Autodesk Fusion 360 part; units mm, degrees
(part 4 of 5)
sketch "Sketch2" plane through (0, 0, 0) normal (0, 0, 1) x (1, 0, 0)
  arc A0 (28.2898, -146.7842) -> (30.0064, -147.0869) centre (30.8779, -137.1249) ccw construction
  arc A1 (9.3424, -112.1265) -> (12.7274, -116.0513) centre (22.2229, -104.4394) ccw construction
  line L0 (9.8518, -167.6702) -> (17.4021, -163.8233) construction
  circle A2 centre (2.1789, -108.5649) radius 3.375 construction
  line L1 (100.4519, -39.9064) -> (12.7274, -116.0513) construction
  line L2 (28.2898, -146.7842) -> (23.615, -145.5316) construction
  arc A3 (30.9564, -136.2283) -> (29.2133, -136.2283) centre (30.0848, -146.1903) ccw construction
  arc A4 (2.3786, -152.7505) -> (5.279, -154.7068) centre (4.371, -152.9248) ccw construction
  arc A5 (100.4519, -39.9064) -> (105.7604, -37.9868) centre (99.4908, -28.9484) ccw construction
  line L3 (18.4399, -134.3914) -> (17.361, -146.7224) construction
  line L4 (22.8776, -144.4785) -> (23.4829, -137.5592) construction
  arc A6 (-11.1082, -168.6356) -> (3.7484, -173.4033) centre (-3.1387, -169.3329) ccw construction
  arc A7 (23.3547, -162.6662) -> (17.4021, -163.8233) centre (22.396, -173.6243) ccw construction
  line L5 (-5.7907, -107.8678) -> (-7.6374, -128.9799)
  arc A8 (-9.2616, -147.5287) -> (-11.8245, -142.975) centre (-13.8718, -147.1253) ccw construction
  line L6 (4.7746, -145.5276) -> (6.1209, -144.398) construction
  line L7 (24.392, -136.6501) -> (29.2133, -136.2283) construction
  arc A9 (-10.9528, -133.0126) -> (-7.6374, -128.9799) centre (-12.2491, -128.5675) ccw
  circle A10 centre (27.1493, -126.0578) radius 1.5 construction
  line L8 (6.9668, -134.7286) -> (5.8373, -133.3824) construction
  line L9 (-9.2616, -147.5287) -> (-11.1082, -168.6356) construction
  arc A11 (22.8776, -144.4785) -> (23.615, -145.5316) centre (23.8738, -144.5656) ccw construction
  circle A12 centre (24.4911, -156.4418) radius 1.5 construction
  arc A13 (7.9279, -124.4303) -> (4.7319, -125.8533) centre (6.7243, -126.0276) ccw construction
  arc A14 (9.8518, -167.6702) -> (3.7484, -173.4033) centre (16.6616, -181.0354) ccw construction
  circle A15 centre (-3.7013, -153.9753) radius 1.5 construction
  arc A16 (9.3424, -112.1265) -> (-5.7907, -107.8678) centre (2.1789, -108.5649) ccw construction
  arc A17 (24.392, -136.6501) -> (23.4829, -137.5592) centre (24.4791, -137.6463) ccw construction
  line L10 (15.7692, -149.4168) -> (5.279, -154.7068) construction
  line L11 (2.3786, -152.7505) -> (2.6542, -149.601) construction
  circle A18 centre (31.9218, -131.7454) radius 1.5 construction
  line L12 (7.9279, -124.4303) -> (17.3401, -131.4615) construction
  circle A19 centre (-3.1387, -169.3329) radius 3.375 construction
  line L13 (4.4564, -129.0028) -> (4.7319, -125.8533) construction
  arc A20 (4.4564, -129.0028) -> (5.8373, -133.3824) centre (10.4336, -129.5257) ccw construction
  circle A21 centre (-1.043, -123.5913) radius 1.5
  spline S0 degree 5 poles (17.3401, -131.4615) (17.4524, -131.5454) (17.6596, -131.7229) (17.9183, -132.0182) (18.171, -132.4622) (18.3701, -133.0729) (18.4504, -133.5889) (18.4644, -133.9863) (18.4517, -134.2556) (18.4399, -134.3914) knots 0 0 0 0 0 0 0.2 0.4 0.6 0.8 1 1 1 1 1 1 construction
  circle A22 centre (30.1786, -151.6693) radius 1.5 construction
  spline S1 degree 5 poles (17.361, -146.7224) (17.3492, -146.8581) (17.3149, -147.1256) (17.232, -147.5145) (17.0634, -148.0088) (16.7613, -148.5756) (16.4353, -148.9689) (16.1293, -149.2149) (15.8944, -149.3537) (15.7692, -149.4168) knots -1 -1 -1 -1 -1 -1 -0.8 -0.6 -0.4 -0.2 0 0 0 0 0 0 construction
  arc A23 (4.7746, -145.5276) -> (2.6542, -149.601) centre (8.6313, -150.1239) ccw construction
  line L14 (-10.9528, -133.0126) -> (-11.8245, -142.975)
  line L15 (6.1209, -144.398) -> (6.9668, -134.7286) construction
  circle A24 centre (2.1789, -108.5649) radius 2
  line L16 (0.1865, -108.3907) -> (-1.6602, -129.5027) construction
  arc A25 (4.317, -130.0255) -> (6.882, -134.5726) centre (8.9303, -130.4201) ccw
  line L17 (6.882, -134.5726) -> (6.0108, -144.535)
  line L18 (-11.3887, -137.9938) -> (6.5439, -139.5619)
  circle A26 centre (2.1789, -108.5649) radius 8
  line L19 (4.317, -130.0255) -> (4.8399, -124.0484)
  spline S2 degree 5 poles (4.8399, -124.0484) (4.8815, -123.5731) (4.9918, -122.6298) (5.2386, -121.2367) (5.7136, -119.4197) (6.5081, -117.2134) (7.2997, -115.51) (7.9954, -114.2779) (8.5094, -113.4794) (8.779, -113.0859) knots 0 0 0 0 0 0 0.2 0.4 0.6 0.8 1 1 1 1 1 1
  line L20 (0, 0) -> (13.2638, -13.2638) construction
  line L21 (0, 0) -> (18.7579, 0) construction
  line L22 (7.566, -5.4447) -> (6.7175, -4.5962)
  arc A27 (6.7175, -4.5962) -> (4.5962, -6.7175) centre (5.6569, -5.6569) ccw
  line L23 (4.5962, -6.7175) -> (5.4447, -7.566)
  arc A28 (5.4447, -7.566) -> (7.566, -5.4447) centre (6.5054, -6.5054) ccw
  line L24 (7.566, -7.566) -> (4.5962, -4.5962) construction
  arc A29 (4.5962, 6.7175) -> (6.7175, 4.5962) centre (5.6569, 5.6569) ccw
  line L25 (5.4447, 7.566) -> (4.5962, 6.7175)
  arc A30 (7.566, 5.4447) -> (5.4447, 7.566) centre (6.5054, 6.5054) ccw
  line L26 (6.7175, 4.5962) -> (7.566, 5.4447)
  arc A31 (-6.7175, 4.5962) -> (-4.5962, 6.7175) centre (-5.6569, 5.6569) ccw
  line L27 (-7.566, 5.4447) -> (-6.7175, 4.5962)
  arc A32 (-5.4447, 7.566) -> (-7.566, 5.4447) centre (-6.5054, 6.5054) ccw
  line L28 (-4.5962, 6.7175) -> (-5.4447, 7.566)
  arc A33 (-4.5962, -6.7175) -> (-6.7175, -4.5962) centre (-5.6569, -5.6569) ccw
  line L29 (-5.4447, -7.566) -> (-4.5962, -6.7175)
  arc A34 (-7.566, -5.4447) -> (-5.4447, -7.566) centre (-6.5054, -6.5054) ccw
  line L30 (-6.7175, -4.5962) -> (-7.566, -5.4447)
  line L31 (0, 0) -> (0, -132.816) construction
  line L32 (-5, -105.0346) -> (-5, -20)
  spline S3 degree 5 poles (-5.7907, -107.8678) (-5.7382, -107.2682) (-5.6366, -106.0687) (-5.4939, -104.2686) (-5.3227, -101.867) (-5.1465, -98.863) (-5.0482, -96.458) (-5.0088, -94.6529) (-5, -93.4489) (-5, -92.8467) knots 0 0 0 0 0 0 0.2 0.4 0.6 0.8 1 1 1 1 1 1
  line L33 (5, -101.0789) -> (5, -20)
  line L34 (0, 24.5) -> (0, 0) construction
  circle A35 centre (0, 21) radius 3.5
  circle A36 centre (-6.5054, 6.5054) radius 3.5
  circle A37 centre (-6.5054, -6.5054) radius 3.5
  line L35 (0, 0) -> (-9, 0) construction
  arc A38 (-9.8421, -5.4488) -> (-9.8421, 5.4488) centre (-27.0494, 0) ccw
  line L36 (-5, -20) -> (5, -20) construction
  arc A39 (-5, -20) -> (-9.1588, -8.7878) centre (-22.1936, -20) ccw
  line L37 (-9.6985, 7.9385) -> (-3.1931, 22.4331)
  line L38 (9.6985, 7.9385) -> (3.1931, 22.4331)
  circle A40 centre (6.5054, 6.5054) radius 3.5
  arc A41 (9.8421, 5.4488) -> (9.8421, -5.4488) centre (27.0494, 0) ccw
  arc A42 (9.1588, -8.7878) -> (5, -20) centre (22.1936, -20) ccw
  circle A43 centre (6.5054, -6.5054) radius 3.5
  circle A44 centre (0, 0) radius 3.8
  circle A45 centre (0, 12) radius 3.75
  line L39 (0.9091, 19.0167) -> (3.409, 13.5625)
  line L40 (-0.9091, 19.0167) -> (-3.409, 13.5625)
  arc A46 (0.9091, 19.0167) -> (-0.9091, 19.0167) centre (0, 18.6) ccw
  spline S4 degree 5 poles (9.9567, -106.6925) (9.5878, -105.1601) (8.8852, -102.0894) (7.9369, -97.465) (6.8666, -91.2667) (5.829, -83.4768) (5.2712, -77.2155) (5.0493, -72.5017) (5, -69.3506) (5, -67.773) knots 0 0 0 0 0 0 0.2 0.4 0.6 0.8 1 1 1 1 1 1
  point P0 (6.5439, -139.5619)
  point P1 (0, 24.5)
  dimension "d3" = 4
  dimension "d4" = -6
  dimension "d5" = 6
  dimension "d6" = 45
  dimension "d8" = 3
  dimension "d9" = 6.5
  dimension "d12" = 4.2
  dimension "d14" = 360
  dimension "d16" = 5
  dimension "d17" = 5
  dimension "d18" = 7
  dimension "d19" = 24.5
  dimension "d20" = 7
  dimension "d21" = 7
  dimension "d22" = 9
  dimension "d23" = 20
  dimension "d24" = 7.5
  dimension "d26" = 12
  dimension "d27" = 1
  constraint concentric A2 A24
  constraint symmetric A8.end L16 L17.end
  constraint symmetric A9.start L16 A25.end
  constraint symmetric L5.end L16 A25.start
  constraint symmetric A9 L16 A25
  constraint midpoint L14 L18.start
  constraint coincident P0 L18.end
  constraint perpendicular L17 L18
  constraint concentric A24 A26
  constraint coincident L5.start A26
  constraint tangent L5 A26
  constraint parallel L13 L19
  constraint coincident A26 S2.end
  constraint tangent A26 S2
  constraint horizontal L21
  constraint coincident L20.start L21.start
  constraint tangent L22 A27
  constraint tangent A27 L23
  constraint parallel L22 L23
  constraint tangent L23 A28
  constraint tangent L22 A28
  constraint midpoint A28 L24.start
  constraint midpoint A27 L24.end
  constraint coincident L20 L24.end
  constraint parallel L20 L24
  constraint perpendicular L21 L31
  constraint coincident A16 L32.start
  constraint parallel L31 L32
  constraint coincident L32 S3.end
  constraint coincident A16 L33.start
  constraint parallel L31 L33
  constraint coincident P1 L34.start
  constraint perpendicular L21 L34
  constraint coincident P1 A35
  constraint concentric A32 A36
  constraint concentric A34 A37
  constraint perpendicular L34 L35
  constraint coincident L35.end A38
  constraint coincident A36 A38.end
  constraint coincident A37 A38.start
  constraint tangent A36 A38
  constraint tangent A37 A38
  constraint horizontal L36
  constraint tangent A37 A39
  constraint coincident A37 A39.end
  constraint tangent L32 A39
  constraint coincident L34 A35.centre
  constraint coincident A36 L37.start
  constraint coincident A35 L37.end
  constraint tangent A35 L37
  constraint tangent A36 L37
  constraint symmetric L32.end L34 L33.end
  constraint symmetric L34 A36 A40
  constraint symmetric L34 A38.start A41.end
  constraint symmetric L34 A38.end A41.start
  constraint symmetric L34 A38 A41
  constraint symmetric L34 A39.end A42.start
  constraint symmetric L34 A39 A42
  constraint symmetric L34 L37.start L38.start
  constraint symmetric L34 L37.end L38.end
  constraint symmetric L34 A37 A43
  constraint coincident L34 A45.centre
  constraint coincident A45 L39.end
  constraint tangent A45 L39
  constraint coincident A45 L40.end
  constraint tangent A45 L40
  constraint tangent L39 A46
  constraint tangent L40 A46
  constraint coincident A26 S4.start
  constraint coincident L33 S4.end
  constraint tangent A26 S4
  measures "d3" diameter of A24
  measures "d5" distance of A25.start L19.end
  measures "d6" angle of L20 L21
  measures "d8" diameter of A27
  measures "d9" distance of L24.end L20.start
  measures "d12" distance of L24.start L24.end
  measures "d16" distance of L31 L32
  measures "d17" distance of L31 L33
  measures "d18" diameter of A35
  measures "d19" distance of L20.start P1
  measures "d20" diameter of A36
  measures "d21" diameter of A37
  measures "d22" distance of L20.start L35.end
  measures "d23" distance of L20.start L36
  measures "d24" diameter of A45
  measures "d26" distance of L20.start A45.centre
  measures "d27" radius of A46
extrude "Extrude1" add sketch "Sketch2" along normal blind 6 contours L5 A9 L14 A25 L17 L18 A26 L19 S2 | A26 L32 S3 | A26 | A26 L32 L33 A35 A36 A37 A38 A39 L37 L38 A40 A41 A42 A43 A45 L39 L40 | A26 L33 S4 | A37 | A43 | A36 | A40 | A35 L39 L40 A46 picked at (0.167, 22.8547)
equation "d9 = ( ( 7.6 / 2 ) * 1 mm ) + 2.7 mm"

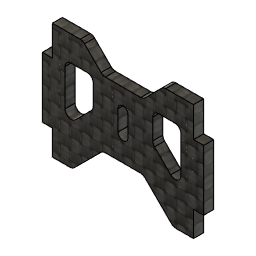
design "cam_mount_2mm"
Autodesk Fusion 360 part; units mm, degrees
sketch "Sketch1" plane through (0, 0, 0) normal (0, 0, 1) x (1, 0, 0)
  line L0 (-16, 11.5) -> (16, 11.5)
  line L1 (16, 11.5) -> (16, -11.5)
  line L2 (16, -11.5) -> (-16, -11.5)
  line L3 (-16, -11.5) -> (-16, 11.5)
  line L4 (-16, 11.5) -> (16, -11.5) construction
  line L5 (16, 11.5) -> (-16, -11.5) construction
  dimension "d1" = 32
  dimension "d2" = 23
  constraint horizontal L0
  constraint perpendicular L0 L1
  constraint parallel L0 L2
  constraint parallel L1 L3
  constraint coincident L4 origin
  constraint coincident L5 origin
  measures "d1" distance of L1.end L2.end
  measures "d2" distance of L0.end L1.end
sketch "Sketch2" plane through (0, 0, 0) normal (0, 0, 1) x (1, 0, 0)
  line L0 (-14, 11.5) -> (14, 11.5)
  line L1 (14, 11.5) -> (14, -11.5)
  line L2 (14, -11.5) -> (-14, -11.5)
  line L3 (-14, -11.5) -> (-14, 11.5)
  line L4 (-14, 11.5) -> (14, -11.5) construction
  line L5 (14, 11.5) -> (-14, -11.5) construction
  line L6 (-16, 5.5) -> (-14, 5.5)
  line L7 (-14, 5.5) -> (-14, -6.5)
  line L8 (-14, -6.5) -> (-16, -6.5)
  line L9 (-16, -6.5) -> (-16, 5.5)
  line L10 (-16, -11.5) -> (-16, 11.5)
  line L11 (-4, 7.5) -> (4, 7.5)
  line L12 (-16, 11.5) -> (16, 11.5)
  line L13 (-4, 7.5) -> (-8, 11.5)
  line L14 (-4, 7.5) -> (0.1526, 7.5) construction
  line L15 (4, 7.5) -> (8, 11.5)
  line L16 (4, 7.5) -> (8.8443, 7.5) construction
  line L17 (0, 0) -> (0, 17.5574) construction
  line L18 (-4, -5.5) -> (4, -5.5)
  line L19 (-4, -5.5) -> (-10, -11.5)
  line L20 (-4, -5.5) -> (4.4853, -5.5) construction
  line L21 (4, -5.5) -> (10, -11.5)
  line L22 (14, 5.5) -> (16, 5.5)
  line L23 (16, 5.5) -> (16, -6.5)
  line L24 (16, -6.5) -> (14, -6.5)
  line L25 (14, -6.5) -> (14, 5.5)
  line L26 (16, 11.5) -> (16, -11.5)
  line L27 (-1, 3.3) -> (-1, -0.7)
  arc A0 (-1, -0.7) -> (1, -0.7) centre (0, -0.7) ccw
  line L28 (1, -0.7) -> (1, 3.3)
  arc A1 (1, 3.3) -> (-1, 3.3) centre (0, 3.3) ccw
  line L29 (0, 4.3) -> (0, -1.7) construction
  line L30 (11.5, 6.5) -> (5.9, 6.5)
  line L31 (5.9, 6.5) -> (5.9, -2.8)
  line L32 (5.9, -2.8) -> (11.5, -2.8)
  line L33 (11.5, -2.8) -> (11.5, 6.5)
  line L34 (5.9, 0.7355) -> (9.4355, -2.8)
  line L35 (5.9, 0.7355) -> (4.4836, 0.7355) construction
  line L36 (11.5, -2.8) -> (11.5, -4.8645)
  line L37 (11.5, -4.8645) -> (9.4355, -2.8)
  point P0 (0, 7.5)
  dimension "d3" = 28
  dimension "d4" = 23
  dimension "d5" = 12
  dimension "d6" = 4
  dimension "d7" = 135
  dimension "d8" = 45
  dimension "d9" = 8
  dimension "d10" = 13
  dimension "d11" = 135
  dimension "d12" = 90
  dimension "d13" = 6
  dimension "d14" = 12
  dimension "d15" = 6
  dimension "d16" = 2
  dimension "d17" = 6
  dimension "d18" = 3.8
  dimension "d19" = 5.6
  dimension "d20" = 9.3
  dimension "d21" = 2.5
  dimension "d22" = 1
  dimension "d23" = 45
  dimension "d24" = 5
  constraint horizontal L0
  constraint perpendicular L0 L1
  constraint parallel L0 L2
  constraint parallel L1 L3
  constraint coincident L4 L17.start
  constraint coincident L5 L17.start
  constraint coincident L17.start origin
  constraint horizontal L6
  constraint vertical L7
  constraint horizontal L8
  constraint vertical L9
  constraint coincident L3 L7.end
  constraint coincident L6.start L10
  constraint horizontal L11
  constraint horizontal L14
  constraint coincident L0 L13.end
  constraint horizontal L16
  constraint coincident L0 L15.end
  constraint vertical L17
  constraint midpoint L11 P0
  constraint coincident L17 P0
  constraint horizontal L20
  constraint coincident L2 L19.end
  constraint coincident L2 L21.end
  constraint horizontal L22
  constraint vertical L23
  constraint horizontal L24
  constraint vertical L25
  constraint coincident L1 L22.start
  constraint coincident L22.end L26
  constraint tangent L27 A0
  constraint tangent A0 L28
  constraint parallel L27 L28
  constraint tangent L28 A1
  constraint tangent L27 A1
  constraint midpoint A1 L29.start
  constraint midpoint A0 L29.end
  constraint parallel L17 L29
  constraint coincident L17 L29.start
  constraint horizontal L30
  constraint vertical L31
  constraint horizontal L32
  constraint vertical L33
  constraint horizontal L35
  constraint coincident L31 L34.start
  constraint coincident L32 L34.end
  constraint perpendicular L32 L36
  constraint parallel L34 L37
  measures "d3" distance of L1.end L2.end
  measures "d4" distance of L0.end L1.end
  measures "d5" distance of L6 L8
  measures "d6" distance of L11 L12
  measures "d7" angle of L13 L14
  measures "d8" angle of L15 L16
  measures "d9" distance of L11.start L11.end
  measures "d11" angle of L19 L20
  measures "d12" angle of L19 L21
  measures "d13" distance of L6 L12
  measures "d14" distance of L22.start L24.end
  measures "d15" distance of L12 L22
  measures "d16" diameter of A0
  measures "d17" distance of L29.start L29.end
  measures "d18" distance of L20 L29.end
  measures "d19" distance of L30.start L30.end
  measures "d20" distance of L30.start L32.end
  measures "d21" distance of L25 L33
  measures "d22" distance of L11 L30
  measures "d23" angle of L34 L35
  measures "d24" distance of L34.start L34.end
extrude "Extrude1" add sketch "Sketch2" along normal blind 2 contours L0 L1 L2 L3 L7 L11 L12 L13 L15 L18 L19 L21 L25 | L3 L6 L7 L8 L9 L10 | L1 L22 L23 L24 L25 L26 | L30 L31 L32 L33 L34 | L32 L36 L37 | L31 L32 L34
extrude "Extrude2" cut sketch "Sketch2" along normal blind 5 contours L30 L31 L32 L33 L34 | L32 L36 L37
fillet "Fillet1" radius 1.2 4 edges at (11.5, -4.8645, 1) (5.9, 0.7355, 1) (5.9, 6.5, 1) (11.5, 6.5, 1)
mirror "Mirror1" about plane through (0, 0, 0) normal (1, 0, 0) of "Extrude2", "Fillet1"
fillet "Fillet2" radius 1.2 8 edges at (-4, -5.5, 1) (-10, -11.5, 1) (4, -5.5, 1) (10, -11.5, 1) (-8, 11.5, 1) (-4, 7.5, 1) (4, 7.5, 1) (8, 11.5, 1)

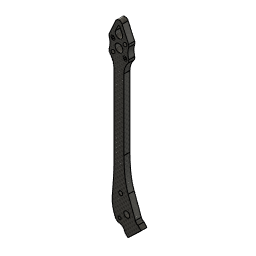
design "arm_rear_6mm"
Autodesk Fusion 360 part; units mm, degrees
sketch "Sketch1" plane through (0, 0, 0) normal (0, 0, 1) x (1, 0, 0)
  circle A0 centre (0, 0) radius 3.95
  line L0 (0, 0) -> (0, -178.3291)
  line L1 (-5, 0) -> (-5, -178.3291)
  line L2 (5, 0) -> (5, -178.3291)
  dimension "d1" = 7.9
  dimension "d2" = 5
  dimension "d3" = -5
  constraint coincident A0.centre L0.start
  constraint vertical L0
  measures "d1" diameter of A0
sketch "Sketch2" plane through (0, 0, 0) normal (0, 0, 1) x (1, 0, 0)
  circle A0 centre (0, 0) radius 3.95
  line L0 (0, 0) -> (-9, 0) construction
  line L1 (7.566, -7.566) -> (4.5962, -4.5962) construction
  line L2 (6.7175, 4.5962) -> (7.566, 5.4447)
  line L3 (4.5962, -6.7175) -> (5.4447, -7.566)
  line L4 (0.9091, 19.0167) -> (3.409, 13.5625)
  circle A1 centre (6.5054, -6.5054) radius 3.5
  line L5 (-4.5962, 6.7175) -> (-5.4447, 7.566)
  arc A2 (4.5962, 6.7175) -> (6.7175, 4.5962) centre (5.6569, 5.6569) ccw
  arc A3 (-7.566, -5.4447) -> (-5.4447, -7.566) centre (-6.5054, -6.5054) ccw
  arc A4 (9.1588, -8.7878) -> (5, -20) centre (22.1936, -20) ccw
  line L6 (7.566, -5.4447) -> (6.7175, -4.5962)
  arc A5 (9.8421, 5.4488) -> (9.8421, -5.4488) centre (27.0494, 0) ccw
  arc A6 (-4.5962, -6.7175) -> (-6.7175, -4.5962) centre (-5.6569, -5.6569) ccw
  circle A7 centre (0, 21) radius 3.5
  circle A8 centre (0, 12) radius 3.75
  line L7 (-5, -20) -> (5, -20) construction
  line L8 (-0.9091, 19.0167) -> (-3.409, 13.5625)
  arc A9 (5.4447, -7.566) -> (7.566, -5.4447) centre (6.5054, -6.5054) ccw
  line L9 (-6.7175, -4.5962) -> (-7.566, -5.4447)
  arc A10 (-5, -20) -> (-9.1588, -8.7878) centre (-22.1936, -20) ccw
  line L10 (5.4447, 7.566) -> (4.5962, 6.7175)
  line L11 (0, 0) -> (18.7579, 0) construction
  circle A11 centre (-6.5054, -6.5054) radius 3.5
  line L12 (-9.6985, 7.9385) -> (-3.1931, 22.4331)
  arc A12 (6.7175, -4.5962) -> (4.5962, -6.7175) centre (5.6569, -5.6569) ccw
  arc A13 (7.566, 5.4447) -> (5.4447, 7.566) centre (6.5054, 6.5054) ccw
  circle A14 centre (-6.5054, 6.5054) radius 3.5
  line L13 (0, 0) -> (13.2638, -13.2638) construction
  line L14 (0, 24.5) -> (0, 0) construction
  line L15 (9.6985, 7.9385) -> (3.1931, 22.4331)
  arc A15 (-6.7175, 4.5962) -> (-4.5962, 6.7175) centre (-5.6569, 5.6569) ccw
  line L16 (-5.4447, -7.566) -> (-4.5962, -6.7175)
  line L17 (-7.566, 5.4447) -> (-6.7175, 4.5962)
  arc A16 (-5.4447, 7.566) -> (-7.566, 5.4447) centre (-6.5054, 6.5054) ccw
  arc A17 (-9.8421, -5.4488) -> (-9.8421, 5.4488) centre (-27.0494, 0) ccw
  circle A18 centre (6.5054, 6.5054) radius 3.5
  arc A19 (0.9091, 19.0167) -> (-0.9091, 19.0167) centre (0, 18.6) ccw
  arc A20 (16.4975, -142.4127) -> (19.1132, -145.1691) centre (20.2426, -141.4781) ccw
  circle A21 centre (28.5466, -163.0999) radius 2.95 construction
  line L18 (36.8072, -178.2122) -> (44.0178, -178.0032) construction
  line L19 (-6.1772, -125.1087) -> (-6.7634, -132.2985)
  line L20 (0.7848, -157.6755) -> (0.9047, -157.0861) construction
  arc A22 (12.4548, -169.2574) -> (12.1429, -164.1911) centre (12.0783, -166.7378) ccw construction
  circle A23 centre (0.6152, -147.9032) radius 1.5
  line L21 (5.9477, -157.6628) -> (12.1429, -164.1911)
  arc A24 (5.9477, -157.6628) -> (0.9047, -157.0861) centre (3.4011, -157.594) ccw
  arc A25 (-7.3343, -135.681) -> (-6.7634, -132.2985) centre (-26.6972, -130.6734) ccw construction
  arc A26 (10.3319, -168.8201) -> (11.86, -169.3463) centre (11.6013, -167.6155) ccw construction
  arc A27 (44.0178, -178.0032) -> (46.9539, -162.6605) centre (43.7859, -170.0066) ccw construction
  arc A28 (36.8072, -178.2122) -> (33.3994, -178.6053) centre (37.3868, -198.2038) ccw construction
  arc A29 (9.2981, -122.9795) -> (-6.1772, -125.1087) centre (1.7963, -125.7587) ccw construction
  line L22 (-7.3343, -135.681) -> (-10.3423, -147.312) construction
  circle A30 centre (21.61, -170.0271) radius 1.5 construction
  line L23 (21.627, -181.0005) -> (33.3994, -178.6053) construction
  arc A31 (0.7848, -157.6755) -> (1.2303, -159.229) centre (2.4997, -158.0244) ccw construction
  line L24 (46.9539, -162.6605) -> (27.9242, -154.4539) construction
  circle A32 centre (1.7963, -125.7587) radius 2
  line L25 (10.3319, -168.8201) -> (1.2303, -159.229) construction
  line L26 (12.4548, -169.2574) -> (11.86, -169.3463) construction
  circle A33 centre (43.7859, -170.0066) radius 2 construction
  line L27 (25.3084, -151.6975) -> (19.1132, -145.1691)
  line L28 (16.4975, -142.4127) -> (9.2981, -122.9795)
  arc A34 (25.3084, -151.6975) -> (27.9242, -154.4539) centre (29.0536, -150.7628) ccw construction
  circle A35 centre (7.8959, -141.3387) radius 2.95
  circle A36 centre (0.6152, -147.9032) radius 4.5
  spline S0 degree 5 poles (0.6152, -152.4032) (0.9218, -152.4032) (1.5117, -152.4518) (2.3269, -152.6706) (3.2887, -153.2145) (4.3168, -154.1801) (5.002, -155.1015) (5.4252, -155.8554) (5.6626, -156.3853) (5.77, -156.657) knots 0 0 0 0 0 0 0.2 0.4 0.6 0.8 1 1 1 1 1 1
  line L29 (22.2108, -148.4333) -> (9.0453, -160.927)
  spline S1 degree 5 poles (-6.7634, -132.2985) (-6.8228, -133.0274) (-6.8958, -134.4803) (-6.8677, -136.6451) (-6.5849, -139.5032) (-5.9007, -143.0251) (-5.105, -145.7887) (-4.35, -147.8195) (-3.7693, -149.1519) (-3.4595, -149.8128) knots 0 0 0 0 0 0 0.2 0.4 0.6 0.8 1 1 1 1 1 1
  line L30 (0, 0) -> (0, -133.0837) construction
  line L31 (-5, 0) -> (-5, -133.0837)
  line L32 (5, 0) -> (5, -133.0837)
  spline S2 degree 5 poles (-6.1772, -125.1087) (-6.1092, -124.2742) (-5.9743, -122.6052) (-5.7752, -120.101) (-5.5198, -116.7611) (-5.2405, -112.5839) (-5.0796, -109.2394) (-5.0145, -106.7287) (-5, -105.0538) (-5, -104.2161) knots 0 0 0 0 0 0 0.2 0.4 0.6 0.8 1 1 1 1 1 1
  spline S3 degree 5 poles (9.2981, -122.9795) (8.8487, -121.7665) (8.0283, -119.3245) (7.033, -115.6132) (6.1133, -110.5828) (5.4305, -104.2105) (5.1351, -99.0813) (5.0246, -95.2302) (5, -92.6623) (5, -91.3783) knots 0 0 0 0 0 0 0.2 0.4 0.6 0.8 1 1 1 1 1 1
  point P0 (0, 24.5)
  dimension "d5" = 360
  dimension "d6" = 45
  dimension "d7" = 3
  dimension "d8" = 6.5
  dimension "d9" = 4.2
  dimension "d10" = 7
  dimension "d11" = 24.5
  dimension "d12" = 7
  dimension "d13" = 7
  dimension "d14" = 9
  dimension "d15" = 20
  dimension "d16" = 7.5
  dimension "d17" = 12
  dimension "d18" = 1
  dimension "d19" = 9
  dimension "d20" = 5
  dimension "d21" = -5
  constraint horizontal L11
  constraint coincident A0.centre L0.start
  constraint tangent L6 A12
  constraint tangent L3 A12
  constraint parallel L3 L6
  constraint tangent L3 A9
  constraint tangent L6 A9
  constraint midpoint L1.start A9
  constraint midpoint L1.end A12
  constraint coincident L1.end L13
  constraint parallel L1 L13
  constraint coincident P0 L14.start
  constraint perpendicular L11 L14
  constraint coincident P0 A7
  constraint concentric A14 A16
  constraint concentric A3 A11
  constraint perpendicular L0 L14
  constraint coincident L0.end A17
  constraint coincident A17.end A14
  constraint coincident A17.start A11
  constraint tangent A14 A17
  constraint tangent A11 A17
  constraint horizontal L7
  constraint tangent A10 A11
  constraint coincident A10.end A11
  constraint coincident A7.centre L14
  constraint coincident L12.start A14
  constraint coincident L12.end A7
  constraint tangent A7 L12
  constraint tangent L12 A14
  constraint symmetric L7.start A4.end L14
  constraint symmetric A14 L14 A18
  constraint symmetric A17.start A5.end L14
  constraint symmetric A17.end A5.start L14
  constraint symmetric A5 L14 A17
  constraint symmetric A10.end A4.start L14
  constraint symmetric A4 A10 L14
  constraint symmetric L12.start L15.start L14
  constraint symmetric L12.end L15.end L14
  constraint symmetric A1 A11 L14
  constraint coincident A8.centre L14
  constraint coincident L4.end A8
  constraint tangent L4 A8
  constraint coincident L8.end A8
  constraint tangent A8 L8
  constraint tangent L4 A19
  constraint tangent L8 A19
  constraint concentric A23 A36
  constraint coincident A36 S0.start
  constraint coincident A24 S0.end
  constraint tangent A24 S0
  constraint tangent A36 S0
  constraint midpoint L27 L29.start
  constraint midpoint L21 L29.end
  constraint coincident A36 S1.end
  constraint tangent A36 S1
  constraint perpendicular L7 L30
  constraint coincident L31 S2.end
  constraint coincident L32 S3.end
  measures "d6" angle of L11 L13
  measures "d7" diameter of A12
  measures "d8" distance of A0.centre L1.end
  measures "d9" distance of L1.start L1.end
  measures "d10" diameter of A7
  measures "d11" distance of P0 A0.centre
  measures "d12" diameter of A14
  measures "d13" diameter of A11
  measures "d14" distance of L0.end A0.centre
  measures "d15" distance of A0.centre L7
  measures "d16" diameter of A8
  measures "d17" distance of A8.centre A0.centre
  measures "d18" radius of A19
  measures "d19" diameter of A36
extrude "Extrude1" add sketch "Sketch2" along normal blind 6 contours L3 A1 A12 L32 | L3 A1 L6 A9 A12 L32 | L4 A1 A5 A7 A8 L8 A11 L12 A14 L15 A17 A18 A20 L19 L21 A24 L27 L28 A36 S0 L29 S1 L31 L32 S2 S3 | A1 A4 L32 | A18 | L4 A7 L8 A19 | A14 | A3 A6 L9 A11 L16 L31 | A10 A11 L31 | A6 A11 L16 L31 | A36 picked at (0.167, 22.8547)

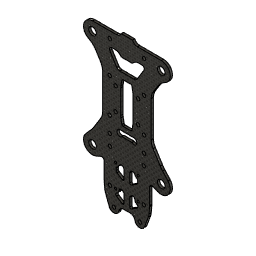
design "mid_plate_2mm"
Autodesk Fusion 360 part; units mm, degrees
sketch "Sketch1" plane through (0, 0, 0) normal (0, 0, 1) x (1, 0, 0)
  line L0 (21.55, -50.4796) -> (21.55, -18.7607)
  line L1 (-21.55, -18.7607) -> (-21.55, -50.4796)
  circle A0 centre (15.25, -19.35) radius 2.95 construction
  circle A1 centre (-15.25, -19.35) radius 2.95 construction
  arc A2 (10.3384, 3) -> (6.0958, 1.2426) centre (10.3384, -3) ccw
  line L2 (-27.7114, -5.7461) -> (-23.2215, -12.9316)
  line L3 (29.5877, -66.4969) -> (23.2215, -56.3087)
  arc A3 (21.55, -50.4796) -> (23.2215, -56.3087) centre (32.55, -50.4796) ccw
  line L4 (4.8532, 0) -> (6.0958, 1.2426)
  circle A4 centre (15, -73.65) radius 2.95 construction
  arc A5 (4.5, -61) -> (8.3897, -57.7389) centre (6.3028, -59.2001) ccw
  line L5 (30.5, 15.05) -> (21.55, 15.05)
  arc A6 (8.0447, -57.2462) -> (6.6112, -56.5) centre (6.6112, -58.25) ccw
  line L6 (-4.5, -79.15) -> (4.5, -79.15) construction
  circle A7 centre (30.5, -79.95) radius 2 construction
  circle A8 centre (15.25, -49.85) radius 2.95 construction
  arc A9 (27.3521, -87.3046) -> (36.4601, -74.6136) centre (30.5, -79.95) ccw
  arc A10 (-8.3897, -57.7389) -> (-4.5, -61) centre (-6.3028, -59.2001) ccw
  arc A11 (-30.5, 15.05) -> (-33.9547, -0.1656) centre (-30.5, 7.05) ccw
  arc A12 (-6.0958, 1.2426) -> (-10.3384, 3) centre (-10.3384, -3) ccw
  line L7 (-27.3521, -87.3046) -> (-20.2, -84.2434)
  arc A13 (-31.6483, -69.2394) -> (-29.5877, -66.4969) centre (-46.5487, -55.8985) ccw
  line L8 (-13.5, 3) -> (-10.3384, 3)
  line L9 (-6.0958, 1.2426) -> (-4.8532, 0)
  line L10 (-31.6483, -69.2394) -> (-36.4601, -74.6136)
  arc A14 (15.1961, -0.0598) -> (13.5, 3) centre (13.5, 1) ccw
  arc A15 (19, 46.9161) -> (14.75, 54.55) centre (14.75, 49.55) ccw construction
  arc A16 (-36.4601, -74.6136) -> (-27.3521, -87.3046) centre (-30.5, -79.95) ccw
  circle A17 centre (-15.25, -49.85) radius 2.95 construction
  arc A18 (-6.6112, -56.5) -> (-8.0447, -57.2462) centre (-6.6112, -58.25) ccw
  line L11 (0.3197, 52.9873) -> (5.4482, 50.7517) construction
  arc A19 (2.7973, 58.6708) -> (-2.7973, 58.6708) centre (0, 52.254) ccw construction
  circle A20 centre (-15, -73.65) radius 2.95 construction
  line L12 (-23.2215, -56.3087) -> (-29.5877, -66.4969)
  arc A21 (18.55, 18.05) -> (21.55, 15.05) centre (21.55, 18.05) ccw construction
  arc A22 (-1.3481, 45.8161) -> (1.3481, 45.8161) centre (0, 47.9215) ccw construction
  arc A23 (33.9547, -0.1656) -> (30.5, 15.05) centre (30.5, 7.05) ccw
  line L13 (6.189, -12.7) -> (-6.189, -12.7) construction
  arc A24 (-13.5, 3) -> (-15.1961, -0.0598) centre (-13.5, 1) ccw
  circle A25 centre (15.25, -63.85) radius 1.5
  arc A26 (8.3, -79.15) -> (4.5, -79.15) centre (6.4, -82.51) ccw construction
  circle A27 centre (15.25, 8.95) radius 1.5
  circle A28 centre (-30.5, 7.05) radius 2 construction
  arc A29 (7.55, 40.0871) -> (5.7029, 41.0977) centre (6.35, 40.0871) ccw construction
  arc A30 (9.75, 29.95) -> (11.75, 29.95) centre (10.75, 29.95) ccw construction
  arc A31 (2.35, 33.9294) -> (3.3622, 32.0776) centre (4.55, 33.9294) ccw construction
  line L14 (10.9121, 55.1332) -> (2.7973, 58.6708) construction
  line L15 (-5.4482, 50.7517) -> (-0.3197, 52.9873) construction
  line L16 (9.75, 29.95) -> (9.75, 41.95) construction
  arc A32 (-13.7095, 54.55) -> (-10.9121, 55.1332) centre (-13.7095, 61.55) ccw construction
  line L17 (4.253, 25.5647) -> (8.8217, 22.262) construction
  line L18 (14.75, 54.55) -> (13.7095, 54.55) construction
  line L19 (6.43, 17.6256) -> (2.818, 20.406) construction
  line L20 (-2.7973, 58.6708) -> (-10.9121, 55.1332) construction
  circle A33 centre (-14.75, 49.55) radius 1.5 construction
  line L21 (9.65, 20.6411) -> (9.65, 19.2104) construction
  line L22 (2.35, 33.9294) -> (2.35, 37.7471) construction
  arc A34 (3.3637, 39.5999) -> (2.35, 37.7471) centre (4.55, 37.7471) ccw construction
  line L23 (-8.8217, 22.262) -> (-4.253, 25.5647) construction
  arc A35 (11.75, 41.95) -> (9.75, 41.95) centre (10.75, 41.95) ccw construction
  arc A36 (-13.55, 35.95) -> (-15.55, 35.95) centre (-14.55, 35.95) ccw construction
  line L24 (18.55, 18.05) -> (18.55, 45.3357) construction
  line L25 (-2.35, 24.5922) -> (-2.35, 21.3569) construction
  line L26 (13.55, 23.95) -> (13.55, 35.95) construction
  arc A37 (15.55, 35.95) -> (13.55, 35.95) centre (14.55, 35.95) ccw construction
  circle A38 centre (14.75, 49.55) radius 1.5 construction
  arc A39 (-2.818, 20.406) -> (-2.35, 21.3569) centre (-3.55, 21.3569) ccw construction
  line L27 (7.55, 40.0871) -> (7.55, 33.4162) construction
  arc A40 (5.6227, 48.5531) -> (5.4482, 50.7517) centre (4.9486, 49.6058) ccw construction
  arc A41 (-2.35, 37.7471) -> (-3.3637, 39.5999) centre (-4.55, 37.7471) ccw construction
  arc A42 (-3.3622, 32.0776) -> (-2.35, 33.9294) centre (-4.55, 33.9294) ccw construction
  arc A43 (4.1622, 31.5645) -> (7.55, 33.4162) centre (5.35, 33.4162) ccw construction
  line L28 (-11.75, 29.95) -> (-11.75, 41.95) construction
  line L29 (-2.818, 20.406) -> (-6.43, 17.6256) construction
  line L30 (-9.75, 41.95) -> (-9.75, 29.95) construction
  line L31 (4.1622, 31.5645) -> (3.3622, 32.0776) construction
  arc A44 (-14.75, 54.55) -> (-19, 46.9161) centre (-14.75, 49.55) ccw construction
  line L32 (11.75, 41.95) -> (11.75, 29.95) construction
  line L33 (-13.7095, 54.55) -> (-14.75, 54.55) construction
  line L34 (-15.55, 23.95) -> (-15.55, 35.95) construction
  arc A45 (-15.55, 23.95) -> (-13.55, 23.95) centre (-14.55, 23.95) ccw construction
  line L35 (5.6227, 48.5531) -> (1.3481, 45.8161) construction
  arc A46 (-7.55, 33.4162) -> (-4.1622, 31.5645) centre (-5.35, 33.4162) ccw construction
  line L36 (-9.65, 19.2104) -> (-9.65, 20.6411) construction
  arc A47 (-2.35, 24.5922) -> (-4.253, 25.5647) centre (-3.55, 24.5922) ccw construction
  line L37 (-1.3481, 45.8161) -> (-5.6227, 48.5531) construction
  arc A48 (-5.7029, 41.0977) -> (-7.55, 40.0871) centre (-6.35, 40.0871) ccw construction
  arc A49 (-18.55, 45.3357) -> (-19, 46.9161) centre (-21.55, 45.3357) ccw construction
  line L38 (-3.3622, 32.0776) -> (-4.1622, 31.5645) construction
  arc A50 (4.253, 25.5647) -> (2.35, 24.5922) centre (3.55, 24.5922) ccw construction
  arc A51 (0.3197, 52.9873) -> (-0.3197, 52.9873) centre (0, 52.254) ccw construction
  arc A52 (19, 46.9161) -> (18.55, 45.3357) centre (21.55, 45.3357) ccw construction
  line L39 (2.35, 21.3569) -> (2.35, 24.5922) construction
  arc A53 (10.9121, 55.1332) -> (13.7095, 54.55) centre (13.7095, 61.55) ccw construction
  line L40 (-13.55, 35.95) -> (-13.55, 23.95) construction
  arc A54 (13.55, 23.95) -> (15.55, 23.95) centre (14.55, 23.95) ccw construction
  line L41 (-2.35, 37.7471) -> (-2.35, 33.9294) construction
  line L42 (-7.55, 33.4162) -> (-7.55, 40.0871) construction
  arc A55 (9.65, 20.6411) -> (8.8217, 22.262) centre (7.65, 20.6411) ccw construction
  arc A56 (-5.4482, 50.7517) -> (-5.6227, 48.5531) centre (-4.9486, 49.6058) ccw construction
  arc A57 (2.35, 21.3569) -> (2.818, 20.406) centre (3.55, 21.3569) ccw construction
  arc A58 (-8.8217, 22.262) -> (-9.65, 20.6411) centre (-7.65, 20.6411) ccw construction
  line L43 (-5.7029, 41.0977) -> (-3.3637, 39.5999) construction
  line L44 (3.3637, 39.5999) -> (5.7029, 41.0977) construction
  line L45 (-18.55, 45.3357) -> (-18.55, 18.05) construction
  line L46 (15.55, 35.95) -> (15.55, 23.95) construction
  arc A59 (-9.75, 41.95) -> (-11.75, 41.95) centre (-10.75, 41.95) ccw construction
  arc A60 (-11.75, 29.95) -> (-9.75, 29.95) centre (-10.75, 29.95) ccw construction
  line L47 (4.5, -61) -> (-4.5, -61)
  arc A61 (6.43, 17.6256) -> (9.65, 19.2104) centre (7.65, 19.2104) ccw construction
  arc A62 (-9.65, 19.2104) -> (-6.43, 17.6256) centre (-7.65, 19.2104) ccw construction
  line L48 (36.4601, -74.6136) -> (31.6483, -69.2394)
  arc A63 (-21.55, 15.05) -> (-18.55, 18.05) centre (-21.55, 18.05) ccw construction
  line L49 (-6.6112, -56.5) -> (6.6112, -56.5)
  line L50 (-21.55, 15.05) -> (-30.5, 15.05)
  line L51 (8.0447, -57.2462) -> (8.3897, -57.7389)
  circle A64 centre (-15.25, 8.95) radius 1.5
  line L52 (8.3, -79.15) -> (27.3521, -87.3046) construction
  arc A65 (29.5877, -66.4969) -> (31.6483, -69.2394) centre (46.5487, -55.8985) ccw
  circle A66 centre (-30.5, -79.95) radius 2 construction
  line L53 (-8.3897, -57.7389) -> (-8.0447, -57.2462)
  arc A67 (-27.7114, -5.7461) -> (-33.9547, -0.1656) centre (-40.4322, -13.6949) ccw
  line L54 (10.3384, 3) -> (13.5, 3)
  arc A68 (23.2215, -12.9316) -> (21.55, -18.7607) centre (32.55, -18.7607) ccw
  arc A69 (-23.2215, -56.3087) -> (-21.55, -50.4796) centre (-32.55, -50.4796) ccw
  arc A70 (-4.5, -79.15) -> (-8.3, -79.15) centre (-6.4, -82.51) ccw construction
  arc A71 (33.9547, -0.1656) -> (27.7114, -5.7461) centre (40.4322, -13.6949) ccw
  arc A72 (-21.55, -18.7607) -> (-23.2215, -12.9316) centre (-32.55, -18.7607) ccw
  circle A73 centre (30.5, 7.05) radius 2 construction
  circle A74 centre (-15.25, -63.85) radius 1.5
  line L55 (-4.8532, 0) -> (4.8532, 0)
  line L56 (23.2215, -12.9316) -> (27.7114, -5.7461)
  line L57 (15.1961, -0.0598) -> (9.0119, -10.0491)
  circle A75 centre (-30.5, 7.05) radius 3.375
  circle A76 centre (30.5, 7.05) radius 3.375
  circle A77 centre (-30.5, -79.95) radius 3.375
  circle A78 centre (30.5, -79.95) radius 3.375
  circle A79 centre (-15.25, -19.35) radius 1.5
  circle A80 centre (15.25, -19.35) radius 1.5
  circle A81 centre (15.25, -49.85) radius 1.5
  circle A82 centre (-15.25, -49.85) radius 1.5
  line L58 (-15.25, -19.35) -> (15.25, -49.85) construction
  line L59 (-10, -24.6) -> (10, -24.6) construction
  line L60 (10, -24.6) -> (10, -44.6) construction
  line L61 (10, -44.6) -> (-10, -44.6) construction
  line L62 (-10, -44.6) -> (-10, -24.6) construction
  line L63 (-10, -24.6) -> (10, -44.6) construction
  line L64 (10, -24.6) -> (-10, -44.6) construction
  circle A83 centre (-10, -24.6) radius 1.5
  circle A84 centre (10, -24.6) radius 1.5
  circle A85 centre (10, -44.6) radius 1.5
  circle A86 centre (-10, -44.6) radius 1.5
  circle A87 centre (-15, -73.65) radius 1.5
  circle A88 centre (15, -73.65) radius 1.5
  line L65 (6.189, -11.4) -> (-6.189, -11.4)
  line L66 (0, 44.45) -> (0, -156.9165) construction
  spline S0 degree 5 poles (9.0119, -10.0491) (8.9382, -10.1683) (8.7794, -10.3902) (8.5077, -10.6735) (8.0875, -10.964) (7.4965, -11.2156) (6.9894, -11.3405) (6.5947, -11.3892) (6.3253, -11.4) (6.189, -11.4) knots 0 0 0 0 0 0 0.2 0.4 0.6 0.8 1 1 1 1 1 1
  line L67 (-15.1961, -0.0598) -> (-9.0119, -10.0491)
  spline S1 degree 5 poles (-9.0119, -10.0491) (-8.9382, -10.1683) (-8.7794, -10.3902) (-8.5077, -10.6735) (-8.0875, -10.964) (-7.4965, -11.2156) (-6.9894, -11.3405) (-6.5947, -11.3892) (-6.3253, -11.4) (-6.189, -11.4) knots 0 0 0 0 0 0 0.2 0.4 0.6 0.8 1 1 1 1 1 1
  line L68 (9.2055, -9.7365) -> (8.8184, -10.3617)
  line L69 (6.5567, -11.4) -> (5.8214, -11.4)
  line L70 (-9.2055, -9.7365) -> (-8.8184, -10.3617)
  line L71 (-6.5567, -11.4) -> (-5.8214, -11.4)
  line L72 (-5.45, -16.7) -> (5.45, -16.7)
  line L73 (5.45, -16.7) -> (5.45, -52.5)
  line L74 (5.45, -52.5) -> (-5.45, -52.5)
  line L75 (-5.45, -52.5) -> (-5.45, -16.7)
  line L76 (-5.45, -16.7) -> (5.45, -52.5) construction
  line L77 (5.45, -16.7) -> (-5.45, -52.5) construction
  line L78 (-5.45, -23.1541) -> (-4.312, -16.7)
  line L79 (-5.45, -23.1541) -> (0.7741, -23.1541) construction
  line L80 (-5.45, -46.0459) -> (-4.312, -52.5)
  line L81 (-5.45, -46.0459) -> (1.3736, -46.0459) construction
  line L82 (-4.312, -16.7) -> (-4.312, -52.5) construction
  line L83 (5.45, -46.0459) -> (4.312, -52.5)
  line L84 (5.45, -23.1541) -> (4.312, -16.7)
  line L85 (-20.2, -84.2434) -> (-20.2, -102.0248)
  line L86 (0, 18) -> (5, 18)
  line L87 (21.55, 15.05) -> (9.313, 15.05)
  arc A89 (5, 18) -> (9.313, 15.05) centre (9.313, 19.6778) ccw
  arc A90 (-9.313, 15.05) -> (-5, 18) centre (-9.313, 19.6778) ccw
  line L88 (-21.55, 15.05) -> (-9.313, 15.05)
  line L89 (0, 18) -> (-5, 18)
  line L90 (-15, -73.65) -> (-15, -103.65) construction
  circle A91 centre (-15, -103.65) radius 1.5
  circle A92 centre (-11.5, -118.65) radius 1.5
  circle A93 centre (-11.5, -118.65) radius 4.5
  line L91 (-15.7286, -120.1891) -> (-19.5733, -109.626)
  line L92 (-15.7286, -120.1891) -> (-5.1118, -120.1891) construction
  line L93 (-19.5733, -109.626) -> (-20.2, -102.0248)
  line L94 (0, -116) -> (-7.863, -116)
  line L95 (20.2, -84.2434) -> (20.2, -102.0248)
  circle A94 centre (15, -103.65) radius 1.5
  circle A95 centre (11.5, -118.65) radius 1.5
  line L96 (19.5733, -109.626) -> (20.2, -102.0248)
  line L97 (15.7286, -120.1891) -> (5.1118, -120.1891) construction
  line L98 (15.7286, -120.1891) -> (19.5733, -109.626)
  line L99 (0, -116) -> (7.863, -116)
  circle A96 centre (11.5, -118.65) radius 4.5
  line L100 (0, 44.45) -> (0, -156.9165) construction
  line L101 (27.3521, -87.3046) -> (20.2, -84.2434)
  point P0 (0, 44.45)
  point P1 (0, -34.6)
  point P2 (0, -34.6)
  point P3 (6.4, -82.51)
  point P4 (15, -103.65)
  dimension "d1" = 6.75
  dimension "d2" = 3
  dimension "d3" = 20
  dimension "d4" = 20
  dimension "d5" = 3
  dimension "d6" = 1.3
  dimension "d7" = 10.9
  dimension "d8" = 35.8
  dimension "d9" = 80
  dimension "d10" = 80
  dimension "d12" = 20.2
  dimension "d13" = 5
  dimension "d14" = 18
  dimension "d15" = 30
  dimension "d16" = 15
  dimension "d17" = 11.5
  dimension "d18" = 9
  dimension "d19" = 110
  dimension "d20" = 55
  constraint midpoint L55 origin
  constraint concentric A11 A75
  constraint concentric A23 A76
  constraint concentric A16 A77
  constraint concentric A7 A78
  constraint equal A77 A78
  constraint equal A76 A77
  constraint equal A75 A76
  constraint concentric A1 A79
  constraint concentric A0 A80
  constraint concentric A8 A81
  constraint concentric A17 A82
  constraint equal A81 A82
  constraint equal A80 A81
  constraint equal A79 A80
  constraint coincident A1.centre A79.centre
  constraint coincident A8.centre A81.centre
  constraint horizontal L59
  constraint perpendicular L59 L60
  constraint parallel L59 L61
  constraint parallel L60 L62
  constraint coincident L63 P2
  constraint coincident L64 P2
  constraint midpoint L58 P2
  constraint coincident L59.start L62.end
  constraint coincident L59.end L60.start
  constraint coincident L60.end L61.start
  constraint coincident L61.end L62.start
  constraint equal A85 A86
  constraint equal A84 A85
  constraint equal A83 A84
  constraint concentric A20 A87
  constraint concentric A4 A88
  constraint equal A87 A88
  constraint equal A81 A87
  constraint coincident P0 L66.start
  constraint perpendicular L59 L66
  constraint midpoint L57.end L68
  constraint midpoint L65.start L69
  constraint symmetric A14.start L66 A24.end
  constraint symmetric L57.end L66 L67.end
  constraint symmetric L65.start L66 L65.end
  constraint symmetric L66 L68.start L70.start
  constraint symmetric L66 L68.end L70.end
  constraint symmetric L66 L69.start L71.start
  constraint symmetric L66 L69.end L71.end
  constraint horizontal L72
  constraint perpendicular L72 L73
  constraint parallel L72 L74
  constraint parallel L73 L75
  constraint coincident L76 P2
  constraint coincident L77 P2
  constraint coincident P2 P1
  constraint horizontal L79
  constraint coincident L75 L78.start
  constraint horizontal L81
  constraint coincident L75 L80.start
  constraint coincident L74 L80.end
  constraint vertical L82
  constraint coincident L72 L78.end
  constraint symmetric L66 L78.start L84.start
  constraint symmetric L66 L78.end L84.end
  constraint symmetric L66 L80.start L83.start
  constraint symmetric L66 L80.end L83.end
  constraint parallel L66 L85
  constraint coincident L85 L7.end
  constraint coincident L66 L86.start
  constraint perpendicular L66 L86
  constraint tangent A21 L87
  constraint perpendicular L21 L87
  constraint horizontal L87
  constraint tangent L87 A89
  constraint symmetric L5.end L66 A63.start
  constraint symmetric L66 L86.start L89.start
  constraint symmetric L66 L86.end A90.end
  constraint symmetric L66 L87.end A90.start
  constraint symmetric L66 A89 A90
  constraint coincident A20.centre A87.centre
  constraint vertical L90
  constraint coincident L90.end A91.centre
  constraint equal A87 A91
  constraint equal A91 A92
  constraint concentric A92 A93
  constraint horizontal L92
  constraint coincident A93 L91.start
  constraint tangent A93 L91
  constraint coincident L66 L94.start
  constraint perpendicular L66 L94
  constraint coincident A93 L94.end
  constraint symmetric A70.centre L66 P3
  constraint symmetric P0 L66 L100.start
  constraint symmetric L100.end L66 L66.end
  constraint symmetric L66 L85.end L95.end
  constraint symmetric L66 L7.end L95.start
  constraint symmetric L66 L90.end P4
  constraint symmetric L66 A91 A94
  constraint symmetric L66 A92 A95
  constraint symmetric L66 A93 A96
  constraint symmetric L66 L91.start L97.start
  constraint symmetric L66 L91.end L96.start
  constraint symmetric L66 L92.end L97.end
  constraint symmetric L66 L94.start L99.start
  constraint symmetric L66 L94.end L99.end
  constraint symmetric L7.start L66 A9.start
  measures "d1" diameter of A75
  measures "d2" diameter of A79
  measures "d3" distance of L60.end L61.end
  measures "d4" distance of L59.end L60.end
  measures "d5" diameter of A83
  measures "d7" distance of L73.end L74.end
  measures "d8" distance of L72.end L73.end
  measures "d9" angle of L78 L79
  measures "d10" angle of L80 L81
  measures "d12" distance of L66 L85
  measures "d13" distance of L86.start L86.end
  measures "d14" distance of L55 L86
  measures "d15" distance of A20.centre L90.end
  measures "d16" vertical distance of L90.end A92.centre
  measures "d17" distance of L66 A92.centre
  measures "d18" diameter of A93
  measures "d19" angle of L91 L92
  measures "d20" distance of L47 L94
extrude "Extrude1" add sketch "Sketch1" along normal blind 2 contours L0 L1 L2 L3 A3 L5 A9 A11 L7 A13 L10 A16 L12 A23 L48 L50 A65 A67 A68 A69 A71 A72 L56 L85 L86 L87 A89 A90 L88 L89 A93 L91 L93 L94 L95 L96 L98 L99 A96 L101 | A96 | A93 | L72 L75 L78 | L72 L73 L84 | L74 L75 L80 | L73 L74 L83
fillet "Fillet1" radius 2 2 edges at (-20.2, -84.2434, 1) (20.2, -84.2434, 1)
fillet "Fillet2" radius 4 2 edges at (7.863, -116, 1) (-7.863, -116, 1)
fillet "Fillet3" radius 10 4 edges at (-19.5733, -109.626, 1) (-20.2, -102.0248, 1) (19.5733, -109.626, 1) (20.2, -102.0248, 1)
fillet "Fillet4" radius 1 4 edges at (-4.312, -16.7, 1) (4.312, -16.7, 1) (4.312, -52.5, 1) (-4.312, -52.5, 1)
fillet "Fillet5" radius 10 4 edges at (-5.45, -23.1541, 1) (5.45, -23.1541, 1) (5.45, -46.0459, 1) (-5.45, -46.0459, 1)